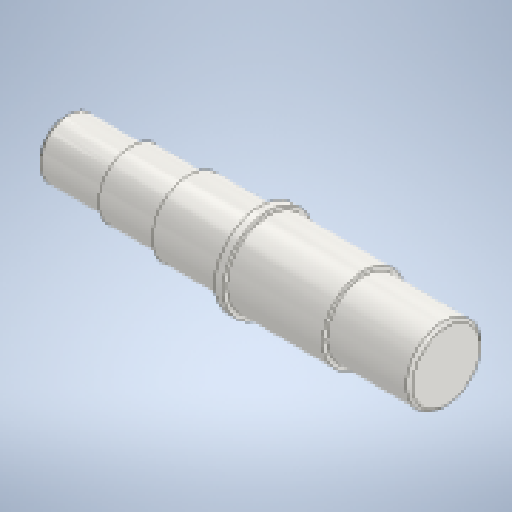
# Autodesk Inventor part: Shaft
Saved by Autodesk Inventor 2025.2 (Build 292293000, 293)
## iProperties
Created: 2024-11-26
Part Number: Shaft
Material: Steel
Document SubType Name: Modeling
Designer: hongquan
Density: 1 g/cm^3
Appearance: Steel
CustomPartVersion: 1
Author: hongquan
Length: 236.000 mm
Autodesk Inventor part; units mm, degrees
ref_plane "Start Plane" through (0, 0, 0) normal (1, 0, 0) x (0, 1, 0)
ref_plane "XZ Plane" through (0, 0, 0) normal (0, 1, 0) x (-1, 0, 0)
ref_plane "XY Plane" through (0, 0, 0) normal (0, 0, 1) x (1, 0, 0)
sketch "Main Sketch" plane through (0, 0, 0) normal (0, 0, 1) x (1, 0, 0)
  line L0 (0, 0) -> (236, 0)
  line L1 (0, 0) -> (0, 17.5)
  line L2 (0, 17.5) -> (45, 17.5)
  line L3 (45, 17.5) -> (45, 20)
  line L4 (45, 20) -> (80, 20)
  line L5 (80, 20) -> (80, 22.5)
  line L6 (80, 22.5) -> (123, 22.5)
  line L7 (123, 22.5) -> (123, 27.5)
  line L8 (128, 27.5) -> (128, 25)
  line L9 (123, 27.5) -> (128, 27.5)
  line L10 (186, 25) -> (186, 22.5)
  line L11 (128, 25) -> (186, 25)
  line L12 (236, 22.5) -> (236, 0)
  line L13 (186, 22.5) -> (236, 22.5)
  dimension "d3" = 35
  dimension "d4" = 40
  dimension "d5" = 45
  dimension "d6" = 55
  dimension "d7" = 50
  dimension "d8" = 45
  constraints: 28 end point, 7 vertical, 4 horizontal
  measures "d3" diameter of L2 L0
  measures "d4" diameter of L4 L0
  measures "d5" diameter of L6 L0
  measures "d6" diameter of L9 L0
  measures "d7" diameter of L11 L0
  measures "d8" diameter of L13 L0
revolve "Revolution1" add sketch "Main Sketch" angle 360 about axis through (0, 0, 0) along (1, 0, 0)
chamfer "Chamfer1" distance 2 angle 45 1 edges at (0, -17.5, 0) measured on face at (30, 17.2734, -2.8072)
chamfer "Chamfer2" distance 2 angle 45 1 edges at (236, -22.5, 0) measured on face at (219.3333, 22.2086, -3.6093)
equation "\"Length\" = 236"
body "Solid1"
